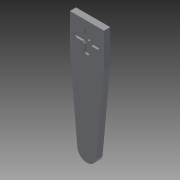
# Autodesk Inventor part: FrontLowerLeg
Saved by Autodesk Inventor 2014 SP1 (Build 180222100, 222)
## iProperties
Created: 2013-09-20
Part Number: FrontLowerLeg
Material: Generic
Document SubType Name: Modeling
Designer: Medrimonia
Density: 1 g/cm^3
Appearance: Default
Author: Medrimonia
Autodesk Inventor part; units mm, degrees
ref_plane "YZ Plane" through (0, 0, 0) normal (1, 0, 0) x (0, 1, 0)
ref_plane "XZ Plane" through (0, 0, 0) normal (0, 1, 0) x (-1, 0, 0)
ref_plane "XY Plane" through (0, 0, 0) normal (0, 0, 1) x (1, 0, 0)
sketch "Sketch1" plane through (0, 0, 0) normal (0, 1, 0) x (-1, 0, 0)
  line L0 (-17.75, -17.75) -> (17.75, -17.75)
  line L1 (17.75, -17.75) -> (17.75, 17.75)
  line L2 (17.75, 17.75) -> (-17.75, 17.75)
  line L3 (-17.75, 17.75) -> (-17.75, -17.75)
  line L4 (-17.75, -17.75) -> (17.75, 17.75) construction
  line L5 (17.75, -17.75) -> (-17.75, 17.75) construction
  line L6 (-2.45, -12.65) -> (2.45, -12.65) construction
  line L7 (2.45, -12.65) -> (2.45, 12.65) construction
  line L8 (2.45, 12.65) -> (-2.45, 12.65) construction
  line L9 (-2.45, 12.65) -> (-2.45, -12.65) construction
  line L10 (-2.45, -12.65) -> (2.45, 12.65) construction
  line L11 (2.45, -12.65) -> (-2.45, 12.65) construction
  line L12 (-12.65, -2.45) -> (12.65, -2.45) construction
  line L13 (12.65, -2.45) -> (12.65, 2.45) construction
  line L14 (12.65, 2.45) -> (-12.65, 2.45) construction
  line L15 (-12.65, 2.45) -> (-12.65, -2.45) construction
  line L16 (-12.65, -2.45) -> (12.65, 2.45) construction
  line L17 (12.65, -2.45) -> (-12.65, 2.45) construction
  line L18 (-12.85, -2.65) -> (12.85, -2.65)
  line L19 (12.85, -2.65) -> (12.85, 2.65)
  line L20 (12.85, 2.65) -> (-12.85, 2.65)
  line L21 (-12.85, 2.65) -> (-12.85, -2.65)
  line L22 (-12.85, -2.65) -> (12.85, 2.65) construction
  line L23 (12.85, -2.65) -> (-12.85, 2.65) construction
  line L24 (-2.65, -12.85) -> (2.65, -12.85)
  line L25 (2.65, -12.85) -> (2.65, 12.85)
  line L26 (2.65, 12.85) -> (-2.65, 12.85)
  line L27 (-2.65, 12.85) -> (-2.65, -12.85)
  line L28 (-2.65, -12.85) -> (2.65, 12.85) construction
  line L29 (2.65, -12.85) -> (-2.65, 12.85) construction
  point P0 (0, 0)
  point P1 (0, 0)
  dimension "d0" = 35.5
  dimension "d1" = 4.9
  dimension "d2" = 10.2
  dimension "d3" = 0.2
  dimension "d4" = 0.2
  constraints: 60 end point, 12 midpoint, 10 parallel, 10 perpendicular, 5 horizontal
  measures "d0" distance of L1.end L2.end
  measures "d1" distance of L14.end L12.start
  measures "d2" distance between parallel lines of L13 L7
  measures "d3" distance between parallel lines of L25 L7
  measures "d4" distance between parallel lines of L26 L8
extrude "Extrusion1" add sketch "Sketch1" along normal blind 1.9
sketch "Sketch2" plane through (0, 1.9, 0) normal (0, 1, 0) x (1, 0, 0)
  line L0 (17.75, 17.75) -> (-17.75, 17.75) projected
  line L1 (-17.75, 17.75) -> (-17.75, -17.75) projected
  line L2 (-17.75, -17.75) -> (17.75, -17.75) projected
  line L3 (17.75, -17.75) -> (17.75, 17.75) projected
  circle A0 centre (0, 0) radius 1.5
  dimension "d7" = 3
  constraints: 1 centre point, 1 coincident
  measures "d7" diameter of A0
extrude "Extrusion2" add sketch "Sketch2" along normal blind 2
sketch "Sketch3" plane through (0, 3.9, 0) normal (0, 1, 0) x (1, 0, 0)
  circle A0 centre (0, 0) radius 1.5 projected
  line L0 (17.75, 17.75) -> (-17.75, 17.75) projected
  line L1 (-17.75, 17.75) -> (-17.75, -17.75) projected
  line L2 (-17.75, -17.75) -> (17.75, -17.75) projected
  line L3 (17.75, -17.75) -> (17.75, 17.75) projected
  circle A1 centre (0, 0) radius 2.75
  dimension "d10" = 5.5
  constraints: 1 centre point, 1 coincident
  measures "d10" diameter of A1
extrude "Extrusion3" add sketch "Sketch3" along normal blind 2.5 contours L3 L2 L1 L0
chamfer "Chamfer1" distance 2 angle 45 1 edges at (-2.65, 0.95, -2.65)
fillet "Fillet1" radius 2.45 1 edges at (-12.85, 0.95, -2.65)
fillet "Fillet2" radius 2.45 1 edges at (-2.65, 0.95, -12.85)
chamfer "Chamfer2" distance 2 angle 45 1 edges at (2.65, 0.95, -2.65)
chamfer "Chamfer3" distance 2 angle 45 1 edges at (2.65, 0.95, 2.65)
fillet "Fillet3" radius 2.45 1 edges at (12.85, 0.95, -2.65)
fillet "Fillet4" radius 2.45 1 edges at (2.65, 0.95, -12.85)
fillet "Fillet5" radius 2.45 1 edges at (12.85, 0.95, 2.65)
fillet "Fillet6" radius 2.45 1 edges at (2.65, 0.95, 12.85)
chamfer "Chamfer4" distance 2 angle 45 1 edges at (-2.65, 0.95, 2.65)
fillet "Fillet7" radius 2.45 2 edges at (-2.65, 0.95, 12.85) (-12.85, 0.95, 2.65)
sketch "Sketch4" plane through (0, 0, 0) normal (0, -1, 0) x (1, 0, 0)
  line L0 (17.75, -17.75) -> (-17.75, -17.75) projected
  line L1 (-10.4, 2.65) -> (-4.65, 2.65) projected
  line L2 (0, 0) -> (0, -74.1645) construction
  line L3 (-17.75, -17.75) -> (-10, -100)
  line L4 (17.75, -17.75) -> (10, -100)
  line L5 (-10, -100) -> (10, -100)
  arc A0 (-10, -100) -> (10, -100) centre (0, -100) ccw
  dimension "d32" = 100
  dimension "d33" = 20
  constraints: 8 end point, 2 perpendicular, 2 point on circle, 1 centre point, 1 midpoint, 1 other
  measures "d32" distance from line of L5 L2.start
  measures "d33" distance of L3.end L4.end
extrude "Extrusion4" add sketch "Sketch4" against normal up to surface (6.4 mm away)
equation "\"d0\" = 3 * ServoArmLength + ServoArmWidth"
equation "\"d1\" = ServoArmWidth"
equation "\"d2\" = ServoArmLength"
equation "\"d3\" = ServoArmSpacing"
equation "\"d4\" = ServoArmSpacing"
equation "\"d5\" = ServoArmThickness"
equation "\"d7\" = ServoArmHoleRequired"
equation "\"d8\" = MinimalThickness"
equation "\"d10\" = ServoArmHeadScrewTrace"
equation "\"d11\" = ServoArmHeadScrewThickness"
equation "\"d13\" = ServoArmInternFillet"
equation "\"d16\" = ServoArmExternFillet"
equation "\"d17\" = ServoArmExternFillet"
equation "\"d18\" = ServoArmInternFillet"
equation "\"d21\" = ServoArmInternFillet"
equation "\"d24\" = ServoArmExternFillet"
equation "\"d25\" = ServoArmExternFillet"
equation "\"d26\" = ServoArmExternFillet"
equation "\"d27\" = ServoArmExternFillet"
equation "\"d28\" = ServoArmInternFillet"
equation "\"d31\" = ServoArmExternFillet"
equation "\"d32\" = FrontLowerLegLength"
equation "\"d33\" = FrontLowerLegFootWidth"
equation "\"d34\" = ServoArmHoleRequired"
equation "\"FrontLowerLegLength\" = 100"
equation "\"FrontLowerLegFootWidth\" = 20"
equation "\"ServoArmLength\" = 10.2"
equation "\"ServoArmWidth\" = 4.9"
equation "\"ServoArmSpacing\" = 0.2"
equation "\"ServoArmThickness\" = 1.9"
equation "\"ServoArmHoleRequired\" = 3"
equation "\"MinimalThickness\" = 2"
equation "\"ServoArmHeadScrewTrace\" = 5.5"
equation "\"ServoArmHeadScrewThickness\" = 2.5"
equation "\"ServoArmInternFillet\" = 2"
equation "\"ServoArmExternFillet\" = 2.45"
body "Solid1"
